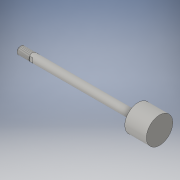
# Autodesk Inventor part: SR-092.5-DPY0_rod
Saved by Autodesk Inventor 2016 SP1 (Build 200210100, 210)
## iProperties
Category: PARTsolutions
Company: BIMBA
Created: 2017-03-09
Part Number: SR-092.5-DPY0_rod
Material: Generic
Catalog Web Link: www.cadenas.de
Description: Standard Air Cylinder_rod-Original Line - Standard Air Cylinders
Vendor: BIMBA
Document SubType Name: Standard Catalog Part
Designer: 589013
Manufacturer: BIMBA
Mass: 18.7068 g
Surface Area: 60.4225 cm^2
Volume: 18.7068 cm^3
Density: 1 g/cm^3
Appearance: PSOLRGB-181-181-181
PSOL_IDENT_0: {$CADENAS_DATA\23d-libs\bimba\bimba\bimba_imperial\bimba_full_line\original_line_cylinders\standard_
PSOL_IDENT_1: air_cylinders\rod.prj},300 {VTYP=3D},{NB=SR-092.5-DPY0_rod},{LINA=SR-092.5-DPY0_rod},{NN=Standard Ai
PSOL_IDENT_2: r Cylinder_rod},{DATE=09.11.2016 07:55:11},{GEOMDATE=10.09.2015 10:40:00},{VERSION=},{LINEID=10},{LI
PSOL_IDENT_3: NESUBID=-1},{WBVAR=STROKE,ACTING,MNT,DER,NR,BM,CO,M,EE,EEL,K,Q,Y,F,G,T,B,H,SER,SR,NT,W,E,HL,ST,STP,P
PSOL_IDENT_4: RC,PB,COLOR1,FCD,RCD,BCD}  {NB=SR-092.5-DPY0_rod},{LINA=SR-092.5-DPY0_rod},{KT=DUMMY},{PN=SR-092.5-D
PSOL_IDENT_5: PY},{DASH=-},{BORE=1.06250000},{BOREPN=09},{STROKE=2.500},{STROKEALG=[0.001:50/0.001]},{STROKE1=2.50
PSOL_IDENT_6: 0},{ACTING=D},{ACTINGALG= '' , 'Single Acting' , 'R' , 'Reverse Single Acting' , 'D' , 'Double Actin
PSOL_IDENT_7: g' },{ACTINGPN=D},{MNT=P},{MNTALG= '' , 'Front Nose Mounting' , 'P' , 'Rear Pivot Mounting' , 'X' , '
PSOL_IDENT_8: Universal Pivot Mounting or Double End Mounting' , 'BF' , 'Front Block Mounting' , 'BR' , 'Rear Bloc
PSOL_IDENT_9: k Mounting for Vertical Positioning' , 'BFT' , 'Front Block Trunnion Mounting' , 'BRT' , 'Rear Block
PSOL_IDENT_10: Trunnion Mounting' },{TYPE=SR-},{MNTPN=P},{DER=},{DERALG= '' , 'N/A' },{NR=},{NRALG= '' , 'N/A' },{
PSOL_IDENT_11: NRPN=},{BM=},{BMALG= '' , 'N/A' },{BMPN=},{CO=},{COALG= '' , 'N/A' },{M=},{MALG= '', 'Without Magnet'
PSOL_IDENT_12: , 'M', 'With Magnet' },{EE=},{EEL=0},{EEMAX=48},{EEALG= '', 'Without Extra Extension', 'EE', 'With E
PSOL_IDENT_13: xtra Extension' },{EELALG=0},{EEPN=},{EEPN1=0.000},{K=},{KALG= '', 'Standard' , 'K' , 'Ports Rotated
PSOL_IDENT_14: 90deg' },{KPN=},{Q=},{QALG= '' , 'Without Side Ported Rear Head' , 'Q' , 'With Side Ported Rear Hea
PSOL_IDENT_15: d' },{QPN=},{Y=Y},{YALG= '' , 'Without Pivot Bushing' , 'Y' , 'With Pivot Bushing' },{YPN=Y},{F=},{F
PSOL_IDENT_16: ALG= '', 'Standard', 'F', 'Molycoated Body' },{FPN=},{G=},{GPN=},{T=},{TALG= '' , 'Standard' , 'N' ,
PSOL_IDENT_17: 'Low Temperature' , 'V' , 'High Temperature' },{NPN=},{VPN=},{B=},{BALG= '', 'Without Bumper' , 'B'
PSOL_IDENT_18: , 'With Bumper' },{BPN=},{H=},{HALG= '', 'N/A' },{HPN=},{SER=},{SERALG= '' , 'Without Spring Extend
PSOL_IDENT_19: /Return' , 'JS' , 'With Spring Return' , 'JR' , 'With Spring Extend' },{SR=SR},{SRALG= 'C' , 'Carbon
PSOL_IDENT_20: Steel Rod' , 'SR' , '303 Stainless Steel Rod' , '' , '303 Stainless Steel Rod1' },{SRPN=SR},{SRCON=
PSOL_IDENT_21: 1},{NT=},{NTPN=},{W=},{WALG= '' , 'Without Wiper' , 'W' , 'With Wiper' },{WPN=},{E=},{EALG= '' , 'Wi
PSOL_IDENT_22: thout Special Lube and Seals' , 'E' , 'With Special Lube and Seals' },{EPN=},{HL=},{HLALG= '' , 'Wih
PSOL_IDENT_23: out Low Pressure Hydraulic' , 'HL' , 'With Low Pressure Hydraulic' },{ST=},{STALG= '' , 'Without Swi
PSOL_IDENT_24: tch Track' , 'T' , 'With Switch Track' },{STP=},{STPALG= '' , 'N/A' },{STPN=},{PRC=},{PRCALG= '' , '
PSOL_IDENT_25: Without Piston Rod Clevis' , 'D-166-1' , 'With Piston Rod Clevis' },{PRCPN=},{PB=},{PBALG= '' , 'Wit
PSOL_IDENT_26: hout Pivot Bracket' , 'D-167' , 'With Pivot Bracket' },{PBPN=},{TLEN=3.8135},{TEXT=0.266667},{SPACE=
PSOL_IDENT_27: 0.152381},{FRAC=10.8400},{RGCON=},{RGDACCON=R},{RHCON=P},{RHCONON=1},{RHACCON=},{FNUTCON=0},{RNUTCON=
PSOL_IDENT_28: 0},{FNUTPN=},{RNUTPN=},{FNUTTRANS=0.0000},{RNUTTRANS=0.0000},{VHOLECON=0},{A1=1.6250},{A1N=1.0000},{
PSOL_IDENT_29: A1P=1.6250},{A1B=1.8750},{A4=0.2525},{A4N=0.3750},{A4P=0.2525},{A5=0.0300},{A1H=1.5},{A1NH=0.6250},{
PSOL_IDENT_30: A1PH=1.5000},{A1BH=1.1250},{A1SH=1.1250},{A2H=0.2500},{A2NH=0.2500},{LENGTH=3.8400},{LENGTH1=3.8400}
PSOL_IDENT_31: ,{LENGTH2=4.1000},{MUL=2.5000},{MUL11=2.5000},{MUL22=6.4000},{MUL33=3.9000},{MUL2=2.5000},{MUL211=2.
PSOL_IDENT_32: 5000},{MUL222=2.5600},{MUL233=1.5600},{SSS=5.0000},{RGLEN=1.4025},{RHLEN=0.9990},{SSS1=3.0000},{A13=
PSOL_IDENT_33: 1.2190},{THDLEN1=0.5000},{THD1=0.3125},{TAB=UNF},{THDLEN=0.5000},{THD=0.3125},{OD=1.0715},{RODL=5.62
PSOL_IDENT_34: 10},{PL=0.8710},{RODDIA=0.3120},{HEX=0.3750},{RODTRANS=0.0000},{G1=0.3440},{ON=0},{G5=0.7180},{DERLE
PSOL_IDENT_35: N=4.6250},{THOLE=0.1900},{WF=0.2500},{BADD=0.0000},{MADD=0.0000},{NVADD=0.000},{JRADD=0.00000},{COLO
PSOL_IDENT_36: R=0.71,0.71,0.71,0.00},{GROOVE=1},{HOL=0},{D7=0.2520},{H1=0.0000},{D1=1.1130},{D1RH=1.1110},{D1P=1.1
PSOL_IDENT_37: 410},{D1B=1.1130},{D1N=1.1130},{D1NRH=1.1155},{D1BRH=1.1410},{D1PRH=1.1110},{BOZO=0},{HADD=0.000},{C
PSOL_IDENT_38: OLOR1=0},{DEFL=0.0000},{HEXL=0.0000},{SSADD=0.0000},{WFL=0.1250},{MOVE=0.1250},{PRCL2=0.50000},{PRCB=
PSOL_IDENT_39: 0.19000},{PRCTRANS=0.19000},{FCD=0},{RCD=0},{BCD=0}
NN: Standard Air Cylinder_rod
NT: Standard
NB: SR-092.5-DPY0_rod
NBSYN: $PN.$COLOR1._rod
LINA: SR-092.5-DPY0_rod
PN: SR-092.5-DPY
BORE: 1.06250000
BOREPN: 09
STROKE: 2.500
ACTING: Double Acting
MNT: Rear Pivot Mounting
DER: N/A
NR: N/A
BM: N/A
CO: N/A
M: Without Magnet
EE: Without Extra Extension
EEL: 0
K: Standard
Q: Without Side Ported Rear Head
Y: With Pivot Bushing
F: Standard
G: Without Magnalube Lubrication
T: Standard
B: Without Bumper
H: N/A
SER: Without Spring Extend/Return
SR: 303 Stainless Steel Rod
W: Without Wiper
E: Without Special Lube and Seals
HL: Wihout Low Pressure Hydraulic
ST: Without Switch Track
STP: N/A
PRC: Without Piston Rod Clevis
PB: Without Pivot Bracket
A1N: 1.0000
A1P: 1.6250
A1B: 1.8750
A4N: 0.3750
A4P: 0.2525
A5: 0.0300
A1NH: 0.6250
A1PH: 1.5000
A1BH: 1.1250
A1SH: 1.1250
A2NH: 0.2500
A13: 1.2190
THDLEN1: 0.5000
THD1: 0.3125
TAB: UNF
OD: 1.0715
RODDIA: 0.3120
HEX: 0.3750
G1: 0.3440
G5: 0.7180
THOLE: 0.1900
WF: 0.2500
GROOVE: 1
D7: 0.2520
D1P: 1.1410
D1B: 1.1130
D1N: 1.1130
D1NRH: 1.1155
D1BRH: 1.1410
D1PRH: 1.1110
COLOR1: 0
FCD: 0
RCD: 0
BCD: 0
SUPPLIER: BIMBA
ARTICLENO: SR-092.5-DPY0_rod
BOMINFO: SR-092.5-DPY0_rod
CREATOR: CADENAS GmbH
Title: SR-092.5-DPY0_rod
Author: Cadenas PARTsolutions
Comments: Original Line - Standard Air Cylinders
Autodesk Inventor part; units mm, degrees
ref_plane "YZ Plane" through (0, 0, 0) normal (1, 0, 0) x (0, 1, 0)
ref_plane "XZ Plane" through (0, 0, 0) normal (0, 1, 0) x (-1, 0, 0)
ref_plane "XY Plane" through (0, 0, 0) normal (0, 0, 1) x (1, 0, 0)
sketch "Sketch_1" plane through (0, 0, 0) normal (0, 0, 1) x (1, 0, 0)
  line L0 (126.8984, 0) -> (-3.175, 0)
  line L1 (-3.175, 0) -> (-3.175, 3.9624)
  line L2 (-3.175, 3.9624) -> (104.775, 3.9624)
  line L3 (104.775, 3.9624) -> (104.775, 13.5572)
  line L4 (104.775, 13.5572) -> (126.8984, 13.5572)
  line L5 (126.8984, 13.5572) -> (126.8984, 0)
  line L6 (126.8984, 0) -> (-3.175, 0)
  constraints: 14 end point
revolve "Revolution1" add sketch "Sketch_1" angle 360 about axis through (126.8984, 0, 0) along (1, 0, 0)
sketch "Sketch_3" plane through (0, 0, 0) normal (0, 0, 1) x (1, 0, 0)
  line L0 (-3.175, 0) -> (-15.875, 0)
  line L1 (-15.875, 0) -> (-15.875, 3.3388)
  line L2 (-15.875, 3.3388) -> (-15.2451, 3.9688)
  line L3 (-15.2451, 3.9688) -> (-3.175, 3.9688)
  line L4 (-3.175, 3.9688) -> (-3.175, 0)
  line L5 (-3.175, 0) -> (-15.875, 0)
  constraints: 12 end point
revolve "Revolution2" add sketch "Sketch_3" angle 360 about axis through (-3.175, 0, 0) along (1, 0, 0)
thread "Thread1" size "5/16-24 UNF" class "2A" standard "ANSI Unified Screw Threads" full length
sketch "Sketch_10" plane through (-3.175, 0, 0) normal (1, 0, 0) x (0, 0, -1)
  line L0 (-7.9248, -7.9248) -> (7.9248, -7.9248)
  line L1 (7.9248, -7.9248) -> (7.9248, 7.9248)
  line L2 (7.9248, 7.9248) -> (-7.9248, 7.9248)
  line L3 (-7.9248, 7.9248) -> (-7.9248, -7.9248)
  line L4 (-3.175, -3.9624) -> (3.175, -3.9624)
  line L5 (3.175, -3.9624) -> (3.175, 3.9624)
  line L6 (3.175, 3.9624) -> (-3.175, 3.9624)
  line L7 (-3.175, 3.9624) -> (-3.175, -3.9624)
  constraints: 16 end point
extrude "Extrusion1" cut sketch "Sketch_10" along normal blind 3.175
ref_plane "dia1_XY" through (-3.175, 3.9624, 0) normal (1, 0, 0) x (0, 0, -1)
ref_plane "dia1_YZ" through (-3.175, 3.9624, 0) normal (0, 0, -1) x (0, 1, 0)
ref_plane "dia1_ZX" through (-3.175, 3.9624, 0) normal (0, 1, 0) x (1, 0, 0)
ref_plane "dia12_XY" through (0, 0, 14.1351) normal (1, 0, 0) x (0, 0, -1)
ref_plane "dia12_YZ" through (0, 0, 14.1351) normal (0, 0, -1) x (0, 1, 0)
ref_plane "dia12_ZX" through (0, 0, 14.1351) normal (0, 1, 0) x (1, 0, 0)
ref_plane "dia2_XY" through (-3.175, -3.9624, 0) normal (1, 0, 0) x (0, 0, -1)
ref_plane "dia2_YZ" through (-3.175, -3.9624, 0) normal (0, 0, -1) x (0, 1, 0)
ref_plane "dia2_ZX" through (-3.175, -3.9624, 0) normal (0, 1, 0) x (1, 0, 0)
ref_plane "dia22_XY" through (0, 0, -14.1351) normal (1, 0, 0) x (0, 0, -1)
ref_plane "dia22_YZ" through (0, 0, -14.1351) normal (0, 0, -1) x (0, 1, 0)
ref_plane "dia22_ZX" through (0, 0, -14.1351) normal (0, 1, 0) x (1, 0, 0)
ref_plane "rl1_XY" through (-15.875, 0, 0) normal (1, 0, 0) x (0, 0, -1)
ref_plane "rl1_YZ" through (-15.875, 0, 0) normal (0, 0, -1) x (0, 1, 0)
ref_plane "rl1_ZX" through (-15.875, 0, 0) normal (0, 1, 0) x (1, 0, 0)
ref_plane "rl2_XY" through (-3.175, 0, 0) normal (1, 0, 0) x (0, 0, -1)
ref_plane "rl2_YZ" through (-3.175, 0, 0) normal (0, 0, -1) x (0, 1, 0)
ref_plane "rl2_ZX" through (-3.175, 0, 0) normal (0, 1, 0) x (1, 0, 0)
ref_plane "rod_cp_XY" through (0, 0, 0) normal (1, 0, 0) x (0, 0, -1)
ref_plane "rod_cp_YZ" through (0, 0, 0) normal (0, 0, -1) x (0, 1, 0)
ref_plane "rod_cp_ZX" through (0, 0, 0) normal (0, 1, 0) x (1, 0, 0)
ref_plane "thd1_XY" through (-15.875, 3.9688, 0) normal (1, 0, 0) x (0, 0, -1)
ref_plane "thd1_YZ" through (-15.875, 3.9688, 0) normal (0, 0, -1) x (0, 1, 0)
ref_plane "thd1_ZX" through (-15.875, 3.9688, 0) normal (0, 1, 0) x (1, 0, 0)
ref_plane "thd2_XY" through (-15.875, -3.9688, 0) normal (1, 0, 0) x (0, 0, -1)
ref_plane "thd2_YZ" through (-15.875, -3.9688, 0) normal (0, 0, -1) x (0, 1, 0)
ref_plane "thd2_ZX" through (-15.875, -3.9688, 0) normal (0, 1, 0) x (1, 0, 0)
ref_plane "to_rod_clevis_XY" through (-20.701, 0, 0) normal (1, 0, 0) x (0, 0, -1)
ref_plane "to_rod_clevis_YZ" through (-20.701, 0, 0) normal (0, 0, -1) x (0, 1, 0)
ref_plane "to_rod_clevis_ZX" through (-20.701, 0, 0) normal (0, 1, 0) x (1, 0, 0)
ref_plane "wf1_XY" through (-3.175, 0, 0) normal (1, 0, 0) x (0, 0, -1)
ref_plane "wf1_YZ" through (-3.175, 0, 0) normal (0, 0, -1) x (0, 1, 0)
ref_plane "wf1_ZX" through (-3.175, 0, 0) normal (0, 1, 0) x (1, 0, 0)
ref_plane "wf2_XY" through (0, 0, 0) normal (1, 0, 0) x (0, 0, -1)
ref_plane "wf2_YZ" through (0, 0, 0) normal (0, 0, -1) x (0, 1, 0)
ref_plane "wf2_ZX" through (0, 0, 0) normal (0, 1, 0) x (1, 0, 0)
ref_plane "wfw1_XY" through (-3.175, 0, -3.175) normal (0, 1, 0) x (1, 0, 0)
ref_plane "wfw1_YZ" through (-3.175, 0, -3.175) normal (1, 0, 0) x (0, 0, -1)
ref_plane "wfw1_ZX" through (-3.175, 0, -3.175) normal (0, 0, -1) x (0, 1, 0)
ref_plane "wfw2_XY" through (-3.175, 0, 3.175) normal (0, 1, 0) x (1, 0, 0)
ref_plane "wfw2_YZ" through (-3.175, 0, 3.175) normal (1, 0, 0) x (0, 0, -1)
ref_plane "wfw2_ZX" through (-3.175, 0, 3.175) normal (0, 0, -1) x (0, 1, 0)
body "Solid1"
